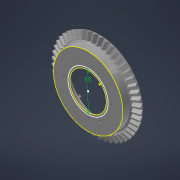
# Autodesk Inventor part: Bevel Gear1
Saved by Autodesk Inventor 2022 (Build 260153000, 153)
## iProperties
CustomPartVersion: 1
Created: 2021-09-12
Part Number: Bevel Gear1
Material: Steel, Mild
Document SubType Name: Modeling
Designer: Andres
Categories: <?xml version="1.0" encoding="UTF-16"?> <MemberInstance><Categories><FamilyTemplate><FamilyTemplateParameter ValueType="xs:double" Id="1" ObjectReferenceKey="da_z" ObjectType="kUserParameterObject"/><FamilyTemplateParameter ValueType="xs:double" Id="2" ObjectReferenceKey="da_b" ObjectType="kUserParameterObject"/><FamilyTemplateParameter ValueType="xs:double" Id="3" ObjectReferenceKey="da_beta" ObjectType="kUserParameterObject"/><FamilyTemplateParameter ValueType="xs:double" Id="4" ObjectReferenceKey="da_dae" ObjectType="kUserParameterObject"/><FamilyTemplateParameter ValueType="xs:double" Id="5" ObjectReferenceKey="da_ve" ObjectType="kUserParameterObject"/><FamilyTemplateParameter ValueType="xs:double" Id="6" ObjectReferenceKey="da_omega" ObjectType="kUserParameterObject"/><FamilyTemplateParameter ValueType="xs:string" Id="7" ObjectReferenceKey="EAIAABAAAAAAHwAAAAAAAIAAAAAAAAAA" ObjectType="83914240" SubObjectId="SurfaceGeometry"/></FamilyTemplate><ParamToTemplateMap><ParamToTemplate CategoryParameter="//CategoryParameter[@InternalName='046C89C9-8512-4d59-83FE-43B91F4F132A']" TemplateParameter="1"/><ParamToTemplate CategoryParameter="//CategoryParameter[@InternalName='2552DF32-E462-4b46-AEBF-C6C7768E72AC']" TemplateParameter="2"/><ParamToTemplate CategoryParameter="//CategoryParameter[@InternalName='C9EE641D-15FC-4fae-A226-E94C4372FDD7']" TemplateParameter="3"/><ParamToTemplate><ParamToTemplate CategoryParameter="//CategoryParameter[@InternalName='00B6519A-459B-49c7-AD84-2E56D39A5744']" ConstantValue="0.000000"/></ParamToTemplate><ParamToTemplate><ParamToTemplate CategoryParameter="//CategoryParameter[@InternalName='04B31F0E-C7A6-4894-AA32-9629BEFACF47']" ConstantValue="1.000000"/></ParamToTemplate><ParamToTemplate><ParamToTemplate CategoryParameter="//CategoryParameter[@InternalName='43CBEC2E-7847-49e7-A936-2F7889FCB2D9']" ConstantValue="0.200000"/></ParamToTemplate><ParamToTemplate><ParamToTemplate CategoryParameter="//CategoryParameter[@InternalName='B1EFC894-105D-4ebd-86BF-FA20ED196853']" ConstantValue="0.300000"/></ParamToTemplate><ParamToTemplate><ParamToTemplate CategoryParameter="//CategoryParameter[@InternalName='51175063-3D10-4879-93E8-6246FE8B403D']" ConstantValue="2060000000.000000"/></ParamToTemplate><ParamToTemplate><ParamToTemplate CategoryParameter="//CategoryParameter[@InternalName='A3A52E27-4454-46a9-B0BD-C932399B70AF']" ConstantValue="0.300000"/></ParamToTemplate><ParamToTemplate CategoryParameter="//CategoryParameter[@InternalName='2A200944-5A8C-41ca-B96E-8520D2E510F1']" TemplateParameter="4"/><ParamToTemplate><ParamToTemplate CategoryParameter="//CategoryParameter[@InternalName='1A637F62-92C8-44bc-B81F-10802510B579']" ConstantValue="10.295893"/></ParamToTemplate><ParamToTemplate CategoryParameter="//CategoryParameter[@InternalName='B52DD4BE-6863-48fb-BF58-89EF6F9EC65C']" TemplateParameter="5"/><ParamToTemplate><ParamToTemplate CategoryParameter="//CategoryParameter[@InternalName='3956BFF2-84D2-457d-93C2-9B0613DEBA67']" ConstantValue="1.810522"/></ParamToTemplate><ParamToTemplate CategoryParameter="//CategoryParameter[@InternalName='739CFA02-461B-4bf8-8049-181FCAD8B28F']" TemplateParameter="6"/><ParamToTemplate><ParamToTemplate CategoryParameter="//CategoryParameter[@InternalName='A27E999F-E2CE-4481-8A2A-EBF499C4C3C5']" ConstantValue="0.000000"/></ParamToTemplate><ParamToTemplate><ParamToTemplate CategoryParameter="//CategoryParameter[@InternalName='9E1B4470-B2D3-4ff1-B813-535BB4CDF51A']" ConstantValue="3300000.000000"/></ParamToTemplate><ParamToTemplate><ParamToTemplate CategoryParameter="//CategoryParameter[@InternalName='F8452263-BFF6-458c-9FB1-07C4B99E95CD']" ConstantValue="3700000.000000"/></ParamToTemplate><ParamToTemplate><ParamToTemplate CategoryParameter="//CategoryParameter[@InternalName='3E3BB259-FD49-497f-8171-6EBC954A3479']" ConstantValue="0.000000"/></ParamToTemplate><ParamToTemplate CategoryParameter="//CategoryParameter[@InternalName='27C3BAF2-7550-4e4b-AE2C-0DB134B7D9B7']" TemplateParameter="7"/></ParamToTemplateMap><Category DisplayName="Gear" InternalName="DC85795E-93AB-48d5-8EEE-5A27447B64BD" Mnemonic="Gear"><CategoryParameter DisplayName="z" InternalName="046C89C9-8512-4d59-83FE-43B91F4F132A" Mnemonic="z"/><CategoryParameter DisplayName="b" InternalName="2552DF32-E462-4b46-AEBF-C6C7768E72AC" Mnemonic="b"/><CategoryParameter DisplayName="||b|" InternalName="C9EE641D-15FC-4fae-A226-E94C4372FDD7" Mnemonic="beta"/><CategoryParameter DisplayName="x" InternalName="00B6519A-459B-49c7-AD84-2E56D39A5744" Mnemonic="x"/><CategoryParameter DisplayName="a*" InternalName="04B31F0E-C7A6-4894-AA32-9629BEFACF47" Mnemonic="a"/><CategoryParameter DisplayName="c*" InternalName="43CBEC2E-7847-49e7-A936-2F7889FCB2D9" Mnemonic="c"/><CategoryParameter DisplayName="r|.f|*" InternalName="B1EFC894-105D-4ebd-86BF-FA20ED196853" Mnemonic="rf"/><CategoryParameter DisplayName="E" InternalName="51175063-3D10-4879-93E8-6246FE8B403D" Mnemonic="E"/><CategoryParameter DisplayName="||m|" InternalName="A3A52E27-4454-46a9-B0BD-C932399B70AF" Mnemonic="mi"/><Category DisplayName="BevelGear" InternalName="0C98F69A-0C2B-4791-B2FE-7691BB227E77" Mnemonic="BevelGear"><CategoryParameter DisplayName="d|.ae|" InternalName="2A200944-5A8C-41ca-B96E-8520D2E510F1" Mnemonic="dae"/><CategoryParameter DisplayName="d|.ai|" InternalName="1A637F62-92C8-44bc-B81F-10802510B579" Mnemonic="dai"/><CategoryParameter DisplayName="A|.e|" InternalName="B52DD4BE-6863-48fb-BF58-89EF6F9EC65C" Mnemonic="ve"/><CategoryParameter DisplayName="A|.i|" InternalName="3956BFF2-84D2-457d-93C2-9B0613DEBA67" Mnemonic="vi"/><CategoryParameter DisplayName="||S|" InternalName="739CFA02-461B-4bf8-8049-181FCAD8B28F" Mnemonic="omega"/><CategoryParameter DisplayName="x|.t|" InternalName="A27E999F-E2CE-4481-8A2A-EBF499C4C3C5" Mnemonic="xt"/><CategoryParameter DisplayName="||s||.Flim|" InternalName="9E1B4470-B2D3-4ff1-B813-535BB4CDF51A" Mnemonic="sFlim"/><CategoryParameter DisplayName="||s||.Hlim|" InternalName="F8452263-BFF6-458c-9FB1-07C4B99E95CD" Mnemonic="sHlim"/><CategoryParameter DisplayName="type" InternalName="3E3BB259-FD49-497f-8171-6EBC954A3479" Mnemonic="type"/><CategoryParameter DisplayName="PitchDiameter" InternalName="27C3BAF2-7550-4e4b-AE2C-0DB134B7D9B7" Mnemonic="IDS_PITCHDIAM"/></Category></Category></Categories></MemberInstance>
Mass: 60.9118 g
Surface Area: 34.3074 cm^2
Volume: 7.7496 cm^3
Density: 7.86 g/cm^3
Appearance: Steel
Author: Andres
Autodesk Inventor part; units mm, degrees
ref_plane "XZ Plane" through (0, 0, 0) normal (0, 1, 0) x (-1, 0, 0)
ref_plane "Mesh Plane2" through (0, 0, 0) normal (0.9978589, 0.0654031, 0) x (0, 0, 1)
sketch "Teeth Body Sketch" plane through (0, 0, 0) normal (1, 0, 0) x (0, 1, 0)
  line L0 (0, 0) -> (58.8959, -26.5394) construction
  line L1 (58.8959, -26.5394) -> (60.9201, -21.4255)
  line L2 (60.9201, -21.4255) -> (0, 0) construction
  line L3 (60, -23.75) -> (0, 0) construction
  line L4 (49.7689, -22.4267) -> (51.4795, -18.1052)
  line L5 (58.8959, -26.5394) -> (49.7689, -22.4267)
  line L6 (60.9201, -21.4255) -> (51.4795, -18.1052)
  line L7 (0, -31.8473) -> (0, 5.3079) projected
  line L8 (0, -23.75) -> (60.9201, -23.75) construction
  dimension "d0" = 120
  dimension "d1" = 117.7917
  dimension "d2" = 121.8402
  dimension "d3" = 10
  dimension "d4" = 21.4255
  constraints: 16 end point, 4 point on line, 3 perpendicular, 2 collinear, 1 horizontal alignment, 1 vertical alignment
  measures "d0" diameter of L3.start L7
  measures "d1" diameter of L0.end L7
  measures "d2" diameter of L1.end L7
  measures "d3" distance between parallel lines of L1 L4
  measures "d4" vertical distance of L1.end L0.start
revolve "Teeth Body" add sketch "Teeth Body Sketch" angle 360 about axis through (0, 0, 0) along (0, 0, 1)
ref_plane "Tooth Plane" through (0, 60, -23.75) normal (0, -0.9298066, 0.3680485) x (1, 0, 0)
sketch "Start Sketch" plane through (0, 60, -23.75) normal (0, -0.9298066, 0.3680485) x (1, 0, 0)
  line L0 (0, -219.1956) -> (0, 51.6432) projected
  arc A0 (-0.7969, -3.66) -> (-3.6705, 4.1097) centre (-55.2032, -19.366) ccw
  arc A1 (3.6705, 4.1097) -> (0.7969, -3.66) centre (55.2032, -19.366) ccw
  line L1 (-0.7969, -3.66) -> (0.7969, -3.66)
  arc A2 (3.6705, 4.1097) -> (-3.6705, 4.1097) centre (0, -163.022) ccw
  dimension "d7" = 56.628
  dimension "d8" = 55.2032
  dimension "d9" = 143.656
  dimension "d57" = 167.172
  dimension "d58" = 159.362
  constraints: 6 point on circle, 3 centre point, 3 symmetric about line, 2 end point, 1 coincident, 1 perpendicular, 1 other
  measures "d7" radius of A0
  measures "d8" horizontal distance of point (0, -163.022) A0.centre
  measures "d9" vertical distance of point (0, -163.022) A0.centre
  measures "d57" radius of A2
  measures "d58" distance from line of A2.centre L1
sketch "End Sketch" plane through (0, 50.4462, -19.9683) normal (0, -0.9298066, 0.3680485) x (1, 0, 0)
  line L0 (0, -187.3249) -> (0, 42.1244) projected
  arc A0 (-0.67, -3.0772) -> (-3.0861, 3.4553) centre (-46.4132, -16.2824) ccw
  arc A1 (3.0861, 3.4553) -> (0.67, -3.0772) centre (46.4132, -16.2824) ccw
  line L1 (-0.67, -3.0772) -> (0.67, -3.0772)
  arc A2 (3.0861, 3.4553) -> (-3.0861, 3.4553) centre (0, -137.0641) ccw
  dimension "d12" = 47.6111
  dimension "d15" = 46.4132
  dimension "d16" = 120.7818
  dimension "d59" = 140.5533
  dimension "d60" = 133.9869
  constraints: 6 point on circle, 3 centre point, 3 symmetric about line, 2 end point, 1 coincident, 1 other
  measures "d12" radius of A0
  measures "d15" horizontal distance of A0.centre point (0, -137.064)
  measures "d16" vertical distance of A0.centre point (0, -137.064)
  measures "d59" radius of A2
  measures "d60" distance from line of A2.centre L1
loft "Loft" cut profiles "Start Sketch", "End Sketch"
pattern_circular "Circular Pattern" count 48 over 360 about axis through (0, 0, 0) along (0, 0, 1) of "Loft"
ref_plane "End Plane" through (0, 50.4462, -19.9683) normal (0, -0.9298066, 0.3680485) x (1, 0, 0)
sketch3d "3D Sketch Right"
ref_plane "End Plane Right" through (-2.7947, 50.3688, -19.9683) normal (0.0515106, -0.9283787, 0.3680485) x (0.9984643, 0.0553993, 0)
sketch "End Sketch Right" plane through (-2.7947, 50.3688, -19.9683) normal (0.0515106, -0.9283787, 0.3680485) x (0.9984643, 0.0553993, 0)
  arc A0 (-0.67, -3.0772) -> (-3.0861, 3.4553) centre (-46.4132, -16.2824) ccw
  line L0 (0, -188.8328) -> (0, 44.5805) projected
  arc A1 (3.0861, 3.4553) -> (0.67, -3.0772) centre (46.4132, -16.2824) ccw
  line L1 (-0.67, -3.0772) -> (0.67, -3.0772)
  arc A2 (3.0861, 3.4553) -> (-3.0861, 3.4553) centre (0, -137.0641) ccw
  dimension "d70" = 46.4132
  dimension "d71" = 120.7818
  dimension "d72" = 47.6111
  dimension "d73" = 133.9869
  dimension "d74" = 140.5533
  constraints: 6 point on circle, 3 centre point, 3 symmetric about line, 2 end point, 1 coincident, 1 perpendicular, 1 other
  measures "d70" horizontal distance of A2.centre A0.centre
  measures "d71" vertical distance of point (0, -137.064) A0.centre
  measures "d72" radius of A0
  measures "d73" distance from line of point (0, -137.064) L1
  measures "d74" radius of A2
feature "Loft Right" [suppressed]
pattern_circular "Circular Pattern Right" [suppressed]
sketch3d "3D Sketch Left"
ref_plane "End Plane Left" through (2.8183, 50.3688, -19.9859) normal (-0.0519386, -0.9282471, 0.3683201) x (0.9984383, -0.0558661, 0)
sketch "End Sketch Left" plane through (2.8183, 50.3688, -19.9859) normal (-0.0519386, -0.9282471, 0.3683201) x (0.9984383, -0.0558661, 0)
  line L0 (0, -188.9711) -> (0, 44.8877) projected
  arc A0 (-0.67, -3.0614) -> (-3.0861, 3.4712) centre (-46.4132, -16.2665) ccw
  arc A1 (3.0861, 3.4712) -> (0.67, -3.0614) centre (46.4132, -16.2665) ccw
  line L1 (-0.67, -3.0614) -> (0.67, -3.0614)
  ellipse E0 centre (0, -16.8324) end of major axis (51.4795, -16.8324) minor radius 18.9609 projected
  arc A2 (3.0861, 3.4712) -> (-3.0861, 3.4712) centre (0, -137.0483) ccw
  dimension "d56" = 18.9609
  dimension "d30" = 47.6111
  dimension "d31" = 46.4132
  dimension "d32" = 120.7818
  dimension "d61" = 140.5533
  dimension "d62" = 133.9869
  constraints: 6 point on circle, 3 centre point, 3 symmetric about line, 2 end point, 1 coincident, 2 other
  measures "d30" radius of A0
  measures "d31" horizontal distance of point (0, -137.048) A0.centre
  measures "d32" vertical distance of A0.centre point (0, -137.048)
  measures "d61" radius of A2
  measures "d62" distance from line of point (0, -137.048) L1
feature "Loft Left" [suppressed]
pattern_circular "Circular Pattern Left" [suppressed]
sketch "Body Sketch" plane through (0, 0, 0) normal (1, 0, 0) x (0, 1, 0)
  line L0 (0, -29.762) -> (0, -7.2041) projected
  line L1 (58.8959, -26.5394) -> (49.7689, -22.4267) projected
  line L2 (49.7689, -22.4267) -> (0, -22.4267)
  line L3 (58.8959, -26.5394) -> (0, -26.5394)
  constraints: 4 end point, 2 perpendicular, 2 point on line
revolve "Fix Body" add sketch "Body Sketch" angle 360 about axis through (0, 0, 0) along (0, 0, 1)
sketch "Sketch6" plane through (0, 0, 0) normal (1, 0, 0) x (0, 1, 0)
  line L0 (60, -23.75) -> (0, 0) projected
  line L1 (0, -31.8473) -> (0, 5.3079) projected
surface revolve "Pitch Diameter" sketch "Sketch6" angle 360 about axis through (0, 0, 0) along (0, 0, 1) shown no curves L0
sketch "Sketch15" plane through (0, 0, -26.5394) normal (0, 0, -1) x (-0.9978589, 0.0654031, 0)
  circle A0 centre (0, 0) radius 25
  arc A1 (4.8399, 58.6966) -> (2.8629, 58.8262) centre (0, 0) ccw projected
  arc A2 (2.8629, 58.8262) -> (-2.8629, 58.8262) centre (0, 0) ccw projected
  arc A3 (-2.8629, 58.8262) -> (-4.8399, 58.6966) centre (0, 0) ccw projected
  arc A4 (-4.8399, 58.6966) -> (-10.5168, 57.9493) centre (0, 0) ccw projected
  arc A5 (-10.5168, 57.9493) -> (-12.46, 57.5628) centre (0, 0) ccw projected
  arc A6 (-12.46, 57.5628) -> (-17.9907, 56.0808) centre (0, 0) ccw projected
  arc A7 (-17.9907, 56.0808) -> (-19.8668, 55.4439) centre (0, 0) ccw projected
  arc A8 (-19.8668, 55.4439) -> (-25.1568, 53.2528) centre (0, 0) ccw projected
  arc A9 (-25.1568, 53.2528) -> (-26.9338, 52.3765) centre (0, 0) ccw projected
  arc A10 (-26.9338, 52.3765) -> (-31.8925, 49.5136) centre (0, 0) ccw projected
  arc A11 (-31.8925, 49.5136) -> (-33.5398, 48.4128) centre (0, 0) ccw projected
  arc A12 (-33.5398, 48.4128) -> (-38.0824, 44.9272) centre (0, 0) ccw projected
  arc A13 (-38.0824, 44.9272) -> (-39.572, 43.6208) centre (0, 0) ccw projected
  arc A14 (-39.572, 43.6208) -> (-43.6208, 39.572) centre (0, 0) ccw projected
  arc A15 (-43.6208, 39.572) -> (-44.9272, 38.0824) centre (0, 0) ccw projected
  arc A16 (-44.9272, 38.0824) -> (-48.4128, 33.5398) centre (0, 0) ccw projected
  arc A17 (-48.4128, 33.5398) -> (-49.5136, 31.8925) centre (0, 0) ccw projected
  arc A18 (-49.5136, 31.8925) -> (-52.3765, 26.9338) centre (0, 0) ccw projected
  arc A19 (-52.3765, 26.9338) -> (-53.2528, 25.1568) centre (0, 0) ccw projected
  arc A20 (-53.2528, 25.1568) -> (-55.4439, 19.8668) centre (0, 0) ccw projected
  arc A21 (-55.4439, 19.8668) -> (-56.0808, 17.9907) centre (0, 0) ccw projected
  arc A22 (-56.0808, 17.9907) -> (-57.5628, 12.46) centre (0, 0) ccw projected
  arc A23 (-57.5628, 12.46) -> (-57.9493, 10.5168) centre (0, 0) ccw projected
  arc A24 (-57.9493, 10.5168) -> (-58.6966, 4.8399) centre (0, 0) ccw projected
  arc A25 (-58.6966, 4.8399) -> (-58.8262, 2.8629) centre (0, 0) ccw projected
  arc A26 (-58.8262, 2.8629) -> (-58.8262, -2.8629) centre (0, 0) ccw projected
  arc A27 (-58.8262, -2.8629) -> (-58.6966, -4.8399) centre (0, 0) ccw projected
  arc A28 (-58.6966, -4.8399) -> (-57.9493, -10.5168) centre (0, 0) ccw projected
  arc A29 (-57.9493, -10.5168) -> (-57.5628, -12.46) centre (0, 0) ccw projected
  arc A30 (-57.5628, -12.46) -> (-56.0808, -17.9907) centre (0, 0) ccw projected
  arc A31 (-56.0808, -17.9907) -> (-55.4439, -19.8668) centre (0, 0) ccw projected
  arc A32 (-55.4439, -19.8668) -> (-53.2528, -25.1568) centre (0, 0) ccw projected
  arc A33 (-53.2528, -25.1568) -> (-52.3765, -26.9338) centre (0, 0) ccw projected
  arc A34 (-52.3765, -26.9338) -> (-49.5136, -31.8925) centre (0, 0) ccw projected
  arc A35 (-49.5136, -31.8925) -> (-48.4128, -33.5398) centre (0, 0) ccw projected
  arc A36 (-48.4128, -33.5398) -> (-44.9272, -38.0824) centre (0, 0) ccw projected
  arc A37 (-44.9272, -38.0824) -> (-43.6208, -39.572) centre (0, 0) ccw projected
  arc A38 (-43.6208, -39.572) -> (-39.572, -43.6208) centre (0, 0) ccw projected
  arc A39 (-39.572, -43.6208) -> (-38.0824, -44.9272) centre (0, 0) ccw projected
  arc A40 (-38.0824, -44.9272) -> (-33.5398, -48.4128) centre (0, 0) ccw projected
  arc A41 (-33.5398, -48.4128) -> (-31.8925, -49.5136) centre (0, 0) ccw projected
  arc A42 (-31.8925, -49.5136) -> (-26.9338, -52.3765) centre (0, 0) ccw projected
  arc A43 (-26.9338, -52.3765) -> (-25.1568, -53.2528) centre (0, 0) ccw projected
  arc A44 (-25.1568, -53.2528) -> (-19.8668, -55.4439) centre (0, 0) ccw projected
  arc A45 (-19.8668, -55.4439) -> (-17.9907, -56.0808) centre (0, 0) ccw projected
  arc A46 (-17.9907, -56.0808) -> (-12.46, -57.5628) centre (0, 0) ccw projected
  arc A47 (-12.46, -57.5628) -> (-10.5168, -57.9493) centre (0, 0) ccw projected
  arc A48 (-10.5168, -57.9493) -> (-4.8399, -58.6966) centre (0, 0) ccw projected
  arc A49 (-4.8399, -58.6966) -> (-2.8629, -58.8262) centre (0, 0) ccw projected
  arc A50 (-2.8629, -58.8262) -> (2.8629, -58.8262) centre (0, 0) ccw projected
  arc A51 (2.8629, -58.8262) -> (4.8399, -58.6966) centre (0, 0) ccw projected
  arc A52 (4.8399, -58.6966) -> (10.5168, -57.9493) centre (0, 0) ccw projected
  arc A53 (10.5168, -57.9493) -> (12.46, -57.5628) centre (0, 0) ccw projected
  arc A54 (12.46, -57.5628) -> (17.9907, -56.0808) centre (0, 0) ccw projected
  arc A55 (17.9907, -56.0808) -> (19.8668, -55.4439) centre (0, 0) ccw projected
  arc A56 (19.8668, -55.4439) -> (25.1568, -53.2528) centre (0, 0) ccw projected
  arc A57 (25.1568, -53.2528) -> (26.9338, -52.3765) centre (0, 0) ccw projected
  arc A58 (26.9338, -52.3765) -> (31.8925, -49.5136) centre (0, 0) ccw projected
  arc A59 (31.8925, -49.5136) -> (33.5398, -48.4128) centre (0, 0) ccw projected
  arc A60 (33.5398, -48.4128) -> (38.0824, -44.9272) centre (0, 0) ccw projected
  arc A61 (38.0824, -44.9272) -> (39.572, -43.6208) centre (0, 0) ccw projected
  arc A62 (39.572, -43.6208) -> (43.6208, -39.572) centre (0, 0) ccw projected
  arc A63 (43.6208, -39.572) -> (44.9272, -38.0824) centre (0, 0) ccw projected
  arc A64 (44.9272, -38.0824) -> (48.4128, -33.5398) centre (0, 0) ccw projected
  arc A65 (48.4128, -33.5398) -> (49.5136, -31.8925) centre (0, 0) ccw projected
  arc A66 (49.5136, -31.8925) -> (52.3765, -26.9338) centre (0, 0) ccw projected
  arc A67 (52.3765, -26.9338) -> (53.2528, -25.1568) centre (0, 0) ccw projected
  arc A68 (53.2528, -25.1568) -> (55.4439, -19.8668) centre (0, 0) ccw projected
  arc A69 (55.4439, -19.8668) -> (56.0808, -17.9907) centre (0, 0) ccw projected
  arc A70 (56.0808, -17.9907) -> (57.5628, -12.46) centre (0, 0) ccw projected
  arc A71 (57.5628, -12.46) -> (57.9493, -10.5168) centre (0, 0) ccw projected
  arc A72 (57.9493, -10.5168) -> (58.6966, -4.8399) centre (0, 0) ccw projected
  arc A73 (58.6966, -4.8399) -> (58.8262, -2.8629) centre (0, 0) ccw projected
  arc A74 (58.8262, -2.8629) -> (58.8262, 2.8629) centre (0, 0) ccw projected
  arc A75 (58.8262, 2.8629) -> (58.6966, 4.8399) centre (0, 0) ccw projected
  arc A76 (58.6966, 4.8399) -> (57.9493, 10.5168) centre (0, 0) ccw projected
  arc A77 (57.9493, 10.5168) -> (57.5628, 12.46) centre (0, 0) ccw projected
  arc A78 (57.5628, 12.46) -> (56.0808, 17.9907) centre (0, 0) ccw projected
  arc A79 (56.0808, 17.9907) -> (55.4439, 19.8668) centre (0, 0) ccw projected
  arc A80 (55.4439, 19.8668) -> (53.2528, 25.1568) centre (0, 0) ccw projected
  arc A81 (53.2528, 25.1568) -> (52.3765, 26.9338) centre (0, 0) ccw projected
  arc A82 (52.3765, 26.9338) -> (49.5136, 31.8925) centre (0, 0) ccw projected
  arc A83 (49.5136, 31.8925) -> (48.4128, 33.5398) centre (0, 0) ccw projected
  arc A84 (48.4128, 33.5398) -> (44.9272, 38.0824) centre (0, 0) ccw projected
  arc A85 (44.9272, 38.0824) -> (43.6208, 39.572) centre (0, 0) ccw projected
  arc A86 (43.6208, 39.572) -> (39.572, 43.6208) centre (0, 0) ccw projected
  arc A87 (39.572, 43.6208) -> (38.0824, 44.9272) centre (0, 0) ccw projected
  arc A88 (38.0824, 44.9272) -> (33.5398, 48.4128) centre (0, 0) ccw projected
  arc A89 (33.5398, 48.4128) -> (31.8925, 49.5136) centre (0, 0) ccw projected
  arc A90 (31.8925, 49.5136) -> (26.9338, 52.3765) centre (0, 0) ccw projected
  arc A91 (26.9338, 52.3765) -> (25.1568, 53.2528) centre (0, 0) ccw projected
  arc A92 (25.1568, 53.2528) -> (19.8668, 55.4439) centre (0, 0) ccw projected
  arc A93 (19.8668, 55.4439) -> (17.9907, 56.0808) centre (0, 0) ccw projected
  arc A94 (17.9907, 56.0808) -> (12.46, 57.5628) centre (0, 0) ccw projected
  arc A95 (12.46, 57.5628) -> (10.5168, 57.9493) centre (0, 0) ccw projected
  arc A96 (10.5168, 57.9493) -> (4.8399, 58.6966) centre (0, 0) ccw projected
  dimension "d137" = 50
  constraints: 1 centre point, 1 coincident
  measures "d137" diameter of A0
sketch "Sketch16" plane through (0, 0, -22.4267) normal (0, 0, 1) x (0.9978589, 0.0654031, 0)
  arc A0 (4.0899, 49.6006) -> (2.4193, 49.7101) centre (0, 0) ccw projected
  arc A1 (2.4193, 49.7101) -> (-2.4193, 49.7101) centre (0, 0) ccw projected
  arc A2 (-2.4193, 49.7101) -> (-4.0899, 49.6006) centre (0, 0) ccw projected
  arc A3 (-4.0899, 49.6006) -> (-8.887, 48.969) centre (0, 0) ccw projected
  arc A4 (-8.887, 48.969) -> (-10.5291, 48.6424) centre (0, 0) ccw projected
  arc A5 (-10.5291, 48.6424) -> (-15.2027, 47.3901) centre (0, 0) ccw projected
  arc A6 (-15.2027, 47.3901) -> (-16.7881, 46.8519) centre (0, 0) ccw projected
  arc A7 (-16.7881, 46.8519) -> (-21.2583, 45.0003) centre (0, 0) ccw projected
  arc A8 (-21.2583, 45.0003) -> (-22.7599, 44.2598) centre (0, 0) ccw projected
  arc A9 (-22.7599, 44.2598) -> (-26.9502, 41.8405) centre (0, 0) ccw projected
  arc A10 (-26.9502, 41.8405) -> (-28.3422, 40.9104) centre (0, 0) ccw projected
  arc A11 (-28.3422, 40.9104) -> (-32.1809, 37.9649) centre (0, 0) ccw projected
  arc A12 (-32.1809, 37.9649) -> (-33.4397, 36.861) centre (0, 0) ccw projected
  arc A13 (-33.4397, 36.861) -> (-36.861, 33.4397) centre (0, 0) ccw projected
  arc A14 (-36.861, 33.4397) -> (-37.9649, 32.1809) centre (0, 0) ccw projected
  arc A15 (-37.9649, 32.1809) -> (-40.9104, 28.3422) centre (0, 0) ccw projected
  arc A16 (-40.9104, 28.3422) -> (-41.8405, 26.9502) centre (0, 0) ccw projected
  arc A17 (-41.8405, 26.9502) -> (-44.2598, 22.7599) centre (0, 0) ccw projected
  arc A18 (-44.2598, 22.7599) -> (-45.0003, 21.2583) centre (0, 0) ccw projected
  arc A19 (-45.0003, 21.2583) -> (-46.8519, 16.7881) centre (0, 0) ccw projected
  arc A20 (-46.8519, 16.7881) -> (-47.3901, 15.2027) centre (0, 0) ccw projected
  arc A21 (-47.3901, 15.2027) -> (-48.6424, 10.5291) centre (0, 0) ccw projected
  arc A22 (-48.6424, 10.5291) -> (-48.969, 8.887) centre (0, 0) ccw projected
  arc A23 (-48.969, 8.887) -> (-49.6006, 4.0899) centre (0, 0) ccw projected
  arc A24 (-49.6006, 4.0899) -> (-49.7101, 2.4193) centre (0, 0) ccw projected
  arc A25 (-49.7101, 2.4193) -> (-49.7101, -2.4193) centre (0, 0) ccw projected
  arc A26 (-49.7101, -2.4193) -> (-49.6006, -4.0899) centre (0, 0) ccw projected
  arc A27 (-49.6006, -4.0899) -> (-48.969, -8.887) centre (0, 0) ccw projected
  arc A28 (-48.969, -8.887) -> (-48.6424, -10.5291) centre (0, 0) ccw projected
  arc A29 (-48.6424, -10.5291) -> (-47.3901, -15.2027) centre (0, 0) ccw projected
  arc A30 (-47.3901, -15.2027) -> (-46.8519, -16.7881) centre (0, 0) ccw projected
  arc A31 (-46.8519, -16.7881) -> (-45.0003, -21.2583) centre (0, 0) ccw projected
  arc A32 (-45.0003, -21.2583) -> (-44.2598, -22.7599) centre (0, 0) ccw projected
  arc A33 (-44.2598, -22.7599) -> (-41.8405, -26.9502) centre (0, 0) ccw projected
  arc A34 (-41.8405, -26.9502) -> (-40.9104, -28.3422) centre (0, 0) ccw projected
  arc A35 (-40.9104, -28.3422) -> (-37.9649, -32.1809) centre (0, 0) ccw projected
  arc A36 (-37.9649, -32.1809) -> (-36.861, -33.4397) centre (0, 0) ccw projected
  arc A37 (-36.861, -33.4397) -> (-33.4397, -36.861) centre (0, 0) ccw projected
  arc A38 (-33.4397, -36.861) -> (-32.1809, -37.9649) centre (0, 0) ccw projected
  arc A39 (-32.1809, -37.9649) -> (-28.3422, -40.9104) centre (0, 0) ccw projected
  arc A40 (-28.3422, -40.9104) -> (-26.9502, -41.8405) centre (0, 0) ccw projected
  arc A41 (-26.9502, -41.8405) -> (-22.7599, -44.2598) centre (0, 0) ccw projected
  arc A42 (-22.7599, -44.2598) -> (-21.2583, -45.0003) centre (0, 0) ccw projected
  arc A43 (-21.2583, -45.0003) -> (-16.7881, -46.8519) centre (0, 0) ccw projected
  arc A44 (-16.7881, -46.8519) -> (-15.2027, -47.3901) centre (0, 0) ccw projected
  arc A45 (-15.2027, -47.3901) -> (-10.5291, -48.6424) centre (0, 0) ccw projected
  arc A46 (-10.5291, -48.6424) -> (-8.887, -48.969) centre (0, 0) ccw projected
  arc A47 (-8.887, -48.969) -> (-4.0899, -49.6006) centre (0, 0) ccw projected
  arc A48 (-4.0899, -49.6006) -> (-2.4193, -49.7101) centre (0, 0) ccw projected
  arc A49 (-2.4193, -49.7101) -> (2.4193, -49.7101) centre (0, 0) ccw projected
  arc A50 (2.4193, -49.7101) -> (4.0899, -49.6006) centre (0, 0) ccw projected
  arc A51 (4.0899, -49.6006) -> (8.887, -48.969) centre (0, 0) ccw projected
  arc A52 (8.887, -48.969) -> (10.5291, -48.6424) centre (0, 0) ccw projected
  arc A53 (10.5291, -48.6424) -> (15.2027, -47.3901) centre (0, 0) ccw projected
  arc A54 (15.2027, -47.3901) -> (16.7881, -46.8519) centre (0, 0) ccw projected
  arc A55 (16.7881, -46.8519) -> (21.2583, -45.0003) centre (0, 0) ccw projected
  arc A56 (21.2583, -45.0003) -> (22.7599, -44.2598) centre (0, 0) ccw projected
  arc A57 (22.7599, -44.2598) -> (26.9502, -41.8405) centre (0, 0) ccw projected
  arc A58 (26.9502, -41.8405) -> (28.3422, -40.9104) centre (0, 0) ccw projected
  arc A59 (28.3422, -40.9104) -> (32.1809, -37.9649) centre (0, 0) ccw projected
  arc A60 (32.1809, -37.9649) -> (33.4397, -36.861) centre (0, 0) ccw projected
  arc A61 (33.4397, -36.861) -> (36.861, -33.4397) centre (0, 0) ccw projected
  arc A62 (36.861, -33.4397) -> (37.9649, -32.1809) centre (0, 0) ccw projected
  arc A63 (37.9649, -32.1809) -> (40.9104, -28.3422) centre (0, 0) ccw projected
  arc A64 (40.9104, -28.3422) -> (41.8405, -26.9502) centre (0, 0) ccw projected
  arc A65 (41.8405, -26.9502) -> (44.2598, -22.7599) centre (0, 0) ccw projected
  arc A66 (44.2598, -22.7599) -> (45.0003, -21.2583) centre (0, 0) ccw projected
  arc A67 (45.0003, -21.2583) -> (46.8519, -16.7881) centre (0, 0) ccw projected
  arc A68 (46.8519, -16.7881) -> (47.3901, -15.2027) centre (0, 0) ccw projected
  arc A69 (47.3901, -15.2027) -> (48.6424, -10.5291) centre (0, 0) ccw projected
  arc A70 (48.6424, -10.5291) -> (48.969, -8.887) centre (0, 0) ccw projected
  arc A71 (48.969, -8.887) -> (49.6006, -4.0899) centre (0, 0) ccw projected
  arc A72 (49.6006, -4.0899) -> (49.7101, -2.4193) centre (0, 0) ccw projected
  arc A73 (49.7101, -2.4193) -> (49.7101, 2.4193) centre (0, 0) ccw projected
  arc A74 (49.7101, 2.4193) -> (49.6006, 4.0899) centre (0, 0) ccw projected
  arc A75 (49.6006, 4.0899) -> (48.969, 8.887) centre (0, 0) ccw projected
  arc A76 (48.969, 8.887) -> (48.6424, 10.5291) centre (0, 0) ccw projected
  arc A77 (48.6424, 10.5291) -> (47.3901, 15.2027) centre (0, 0) ccw projected
  arc A78 (47.3901, 15.2027) -> (46.8519, 16.7881) centre (0, 0) ccw projected
  arc A79 (46.8519, 16.7881) -> (45.0003, 21.2583) centre (0, 0) ccw projected
  arc A80 (45.0003, 21.2583) -> (44.2598, 22.7599) centre (0, 0) ccw projected
  arc A81 (44.2598, 22.7599) -> (41.8405, 26.9502) centre (0, 0) ccw projected
  arc A82 (41.8405, 26.9502) -> (40.9104, 28.3422) centre (0, 0) ccw projected
  arc A83 (40.9104, 28.3422) -> (37.9649, 32.1809) centre (0, 0) ccw projected
  arc A84 (37.9649, 32.1809) -> (36.861, 33.4397) centre (0, 0) ccw projected
  arc A85 (36.861, 33.4397) -> (33.4397, 36.861) centre (0, 0) ccw projected
  arc A86 (33.4397, 36.861) -> (32.1809, 37.9649) centre (0, 0) ccw projected
  arc A87 (32.1809, 37.9649) -> (28.3422, 40.9104) centre (0, 0) ccw projected
  arc A88 (28.3422, 40.9104) -> (26.9502, 41.8405) centre (0, 0) ccw projected
  arc A89 (26.9502, 41.8405) -> (22.7599, 44.2598) centre (0, 0) ccw projected
  arc A90 (22.7599, 44.2598) -> (21.2583, 45.0003) centre (0, 0) ccw projected
  arc A91 (21.2583, 45.0003) -> (16.7881, 46.8519) centre (0, 0) ccw projected
  arc A92 (16.7881, 46.8519) -> (15.2027, 47.3901) centre (0, 0) ccw projected
  arc A93 (15.2027, 47.3901) -> (10.5291, 48.6424) centre (0, 0) ccw projected
  arc A94 (10.5291, 48.6424) -> (8.887, 48.969) centre (0, 0) ccw projected
  arc A95 (8.887, 48.969) -> (4.0899, 49.6006) centre (0, 0) ccw projected
  circle A96 centre (0, 0) radius 47.5
  dimension "d138" = 95
  constraints: 1 centre point, 1 coincident
  measures "d138" diameter of A96
extrude "Extrusion6" add sketch "Sketch16" along normal blind 12 contours A96
chamfer "Chamfer3" distance 2 angle 45 1 edges at (-47.3983, -3.1066, -22.4267)
sketch "Sketch17" plane through (0, 0, -26.5394) normal (0, 0, -1) x (-0.9978589, 0.0654031, 0)
  point P0 (0, 0)
extrude "Extrusion7" cut sketch "Sketch15" against normal through all contours A0
sketch "Sketch18" plane through (0, 0, -26.5394) normal (0, 0, -1) x (-0.9978589, 0.0654031, 0)
  circle A0 centre (0, 0) radius 41 projected
  circle A1 centre (0, 0) radius 30 projected
  circle A2 centre (0, 0) radius 25 projected
  point P0 (0, 0)
extrude "Extrusion8" cut sketch "Sketch18" against normal blind 10 contours A0 | A1 | A2
chamfer "Chamfer4" distance 5 angle 45 1 edges at (40.9122, -2.6815, -16.5394)
chamfer "Chamfer6" distance 5 angle 45 1 edges at (24.9465, -1.6351, -16.5394)
sketch "Sketch20" plane through (0, 0, -16.5394) normal (0, 0, -1) x (-1, 0, 0)
  circle A0 centre (0, 0) radius 32.5 construction
  point P0 (0, 0)
  point P1 (-32.5, 0)
  point P2 (-16.25, -28.1458)
  point P3 (16.25, -28.1458)
  point P4 (32.5, 0)
  point P5 (16.25, 28.1458)
  point P6 (-16.25, 28.1458)
  dimension "d159" = 65
  dimension "d162" = 360
  constraints: 2 horizontal alignment, 1 coincident, 9 other
hole "Hole3" at (-16.25, -28.1458, -16.5394) at (-32.5, 0, -16.5394) at (-16.25, 28.1458, -16.5394) at (16.25, 28.1458, -16.5394) at (32.5, 0, -16.5394) at (16.25, -28.1458, -16.5394) direction (0, 0, 1) diameter 3.242 depth 8 tip angle 118 thread size "M4x0.7" class "6H" standard "ISO Metric profile"
sketch "Sketch21" plane through (0, 0, -10.4267) normal (0, 0, 1) x (1, 0, 0)
  circle A0 centre (0, 0) radius 27.5
  circle A1 centre (0, 0) radius 25 projected
  circle A2 centre (0, 0) radius 47.5 projected
  dimension "d171" = 55
  constraints: 1 centre point, 1 coincident
  measures "d171" diameter of A0
equation "\"d0\" = da_de"
equation "\"d1\" = da_dfe"
equation "\"d2\" = da_dae"
equation "\"d3\" = da_b"
equation "\"d4\" = da_ve"
equation "\"d7\" = fd_rr"
equation "\"d8\" = fd_x"
equation "\"d9\" = fd_y"
equation "\"d57\" = 0.5 * fd_dva + 0.3 * da_he"
equation "\"d58\" = 0.5 * fd_dva - 1.12 * da_he"
equation "\"da_teethtype\" = 0"
equation "\"da_b\" = 10"
equation "\"da_de\" = 120"
equation "\"da_dae\" = 121.84024"
equation "\"da_dfe\" = 117.79171"
equation "\"da_le\" = 64.52955"
equation "\"da_omega\" = 90deg"
equation "\"da_beta\" = 0"
equation "\"da_delta\" = 68.40469deg"
equation "\"da_alpha\" = 20deg"
equation "\"da_he\" = 5.5"
equation "\"da_ve\" = 21.42548"
equation "\"da_zv\" = 130.417612"
equation "\"fd_loft\" = da_b + 0.05 * da_he"
equation "\"fd_x\" = fd_x1 + fd_x2"
equation "\"fd_y\" = fd_y1 - fd_y2"
equation "\"fd_dd\" = fd_dva - 0.8 * da_he"
equation "\"da_dvw\" = 326.04403"
equation "\"d11\" = fd_loft"
equation "\"da_dm\" = 110.70193"
equation "\"da_x\" = 0"
equation "\"da_m\" = 2.5"
equation "\"d50\" = da_omega"
equation "\"fd_rr\" = 56.627956"
equation "\"fd_dva\" = 331.044029"
equation "\"fd_x1\" = 1.985263"
equation "\"fd_x2\" = 53.217962"
equation "\"fd_y1\" = 163.009926"
equation "\"fd_y2\" = 19.353913"
body "Solid1"
body "Srf1"
